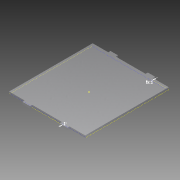
# Autodesk Inventor part: TopPanel
Saved by Autodesk Inventor 2015 SP1 (Build 190203100, 203)
## iProperties
Created: 2015-01-22
Part Number: TopPanel
Material: Acrylic, Clear
Document SubType Name: Modeling
Designer: Patrick
Density: 1.19 g/cm^3
Appearance: Transparent - Clear
Author: Patrick
Autodesk Inventor part; units mm, degrees
ref_plane "YZ Plane" through (0, 0, 0) normal (1, 0, 0) x (0, 1, 0)
ref_plane "XZ Plane" through (0, 0, 0) normal (0, 1, 0) x (-1, 0, 0)
sketch "Sketch1" plane through (0, 0, 0) normal (0, 0, 1) x (1, 0, 0)
  line L0 (-51, 56) -> (51, 56)
  line L1 (51, 56) -> (51, -56)
  line L2 (51, -56) -> (-51, -56)
  line L3 (-51, -56) -> (-51, 56)
  line L4 (-51, 56) -> (51, -56) construction
  line L5 (51, 56) -> (-51, -56) construction
  point P0 (0, 0)
  point P1 (0, 0)
  point P2 (0, 0)
  dimension "d0" = 102
  dimension "d1" = 112
  constraints: 12 end point, 3 midpoint, 2 parallel, 1 coincident, 1 horizontal, 1 perpendicular
  measures "d0" distance of L1.end L2.end
  measures "d1" distance of L0.end L1.end
extrude "Extrusion1" add sketch "Sketch1" along normal blind 3
sketch "Sketch2" plane through (0, 0, 3) normal (0, 0, 1) x (1, 0, 0)
  line L0 (-51, -56) -> (51, -56) projected
  line L1 (-30.065, -59) -> (-19.935, -59)
  line L2 (-19.935, -59) -> (-19.935, -56)
  line L3 (-19.935, -56) -> (-30.065, -56)
  line L4 (-30.065, -56) -> (-30.065, -59)
  line L5 (-30.065, -59) -> (-19.935, -56) construction
  line L6 (-19.935, -59) -> (-30.065, -56) construction
  line L7 (19.935, -59) -> (30.065, -59)
  line L8 (30.065, -59) -> (30.065, -56)
  line L9 (30.065, -56) -> (19.935, -56)
  line L10 (19.935, -56) -> (19.935, -59)
  line L11 (19.935, -59) -> (30.065, -56) construction
  line L12 (30.065, -59) -> (19.935, -56) construction
  point P0 (0, 0)
  point P1 (-25, -57.5)
  point P2 (25, -57.5)
  dimension "d4" = 3
  dimension "d5" = 25
  dimension "d6" = 25
  dimension "d7" = 10.13
  dimension "d8" = 10.13
  constraints: 24 end point, 4 midpoint, 4 parallel, 2 horizontal, 2 perpendicular, 2 point on line, 1 collinear
  measures "d4" distance of L3.end L1.start
  measures "d5" horizontal distance of point (0, 0) point (-25, -57.5)
  measures "d6" horizontal distance of point (25, -57.5) point (0, 0)
  measures "d7" distance of L1.start L1.end
  measures "d8" distance of L7.start L7.end
extrude "Extrusion2" add sketch "Sketch2" against normal blind 3
mirror "Mirror1" about plane through (0, 0, 0) normal (0, 1, 0) of "Extrusion2"
sketch "Sketch3" plane through (0, 0, 0) normal (0, 0, -1) x (-1, 0, 0)
  line L0 (-51, -56) -> (-51, 56) construction
  line L1 (-51, 55) -> (51, 55) construction
  line L2 (51, 56) -> (51, -56) construction
  line L3 (-51, -55) -> (51, -55) construction
  line L4 (-19.935, -56) -> (19.935, -56) construction
  line L5 (-30.065, 56) -> (-51, 56) construction
  point P0 (0, 0)
  dimension "d11" = 1
  dimension "d12" = 1
  constraints: 4 end point, 4 point on line, 1 horizontal, 1 perpendicular
  measures "d11" distance between parallel lines of L4 L3
  measures "d12" distance between parallel lines of L5 L1
ref_plane "Work Plane1" through (-19.935, -55, 0) normal (0, -1, 0) x (1, 0, 0)
sketch "Sketch6" plane through (0, 0, 3) normal (0, 0, 1) x (1, 0, 0)
  line L0 (30.065, -56) -> (51, -56) projected
  line L1 (51, -56) -> (51, 56) projected
  point P0 (0, 0)
  point P1 (20.6, -36.4)
  dimension "d41" = 19.6
  dimension "d42" = 30.4
  measures "d41" distance from line of L0 point (20.6, -36.4)
  measures "d42" distance from line of L1 point (20.6, -36.4)
hole "Hole4" [suppressed]
pattern_linear "Rectangular Pattern1" [suppressed]
sketch "Sketch7" plane through (0, 0, 3) normal (0, 0, 1) x (1, 0, 0)
  spline S0 degree 3 poles (-17.7549, 22.0592) (-20.3586, 22.7486) (-27.8891, 27.7258) (-21.8129, 49.2984) knots 3 3 3 3 4 4 4 4
  line L0 (-20.3586, 22.7486) -> (-27.8891, 27.7258) construction
  line L1 (-17.7549, 22.0592) -> (-20.3586, 22.7486) construction
  line L2 (-27.8891, 27.7258) -> (-21.8129, 49.2984) construction
  spline S1 degree 3 poles (-35.4301, 25.2372) (-34.47, 24.8476) (-28.6027, 22.0592) (-17.7549, 22.0592) knots 2 2 2 2 3 3 3 3
  line L3 (-35.4301, 25.2372) -> (-34.47, 24.8476) construction
  line L4 (-34.47, 24.8476) -> (-28.6027, 22.0592) construction
  line L5 (-28.6027, 22.0592) -> (-17.7549, 22.0592) construction
  spline S2 degree 3 poles (-41.3451, 44.549) (-42.3928, 42.443) (-47.2601, 32.6596) (-35.4301, 25.2372) knots 1 1 1 1 2 2 2 2
  line L6 (-41.3451, 44.549) -> (-42.3928, 42.443) construction
  line L7 (-42.3928, 42.443) -> (-47.2601, 32.6596) construction
  line L8 (-47.2601, 32.6596) -> (-35.4301, 25.2372) construction
  spline S3 degree 3 poles (-37.458, 43.3832) (-40.0894, 43.0815) (-41.2381, 43.3832) (-41.3451, 44.549) knots 0 0 0 0 1 1 1 1
  line L9 (-40.0894, 43.0815) -> (-41.2381, 43.3832) construction
  line L10 (-37.458, 43.3832) -> (-40.0894, 43.0815) construction
  line L11 (-41.2381, 43.3832) -> (-41.3451, 44.549) construction
  spline S4 degree 3 poles (-21.8129, 49.2984) (-21.8202, 49.2933) (-29.1299, 44.232) (-37.458, 43.3832) knots 4 4 4 4 5 5 5 5
  line L12 (-21.8129, 49.2984) -> (-29.1299, 44.232) construction
  line L13 (-29.1299, 44.232) -> (-37.458, 43.3832) construction
  spline S5 degree 3 poles (-15.7483, 21.8123) (-16.0581, 21.8979) (-29.0611, 22.4788) (-21.0119, 50.2568) knots 3 3 3 3 4 4 4 4
  line L14 (-15.7483, 21.8123) -> (-16.0581, 21.8979) construction
  line L15 (-16.0581, 21.8979) -> (-29.0611, 22.4788) construction
  line L16 (-29.0611, 22.4788) -> (-21.0119, 50.2568) construction
  spline S6 degree 3 poles (-21.0119, 50.2568) (-21.2194, 50.1207) (-29.151, 44.9225) (-36.6832, 43.8886) knots 4 4 4 4 5 5 5 5
  line L17 (-21.0119, 50.2568) -> (-21.2194, 50.1207) construction
  line L18 (-21.2194, 50.1207) -> (-29.151, 44.9225) construction
  line L19 (-29.151, 44.9225) -> (-36.6832, 43.8886) construction
  line L20 (-36.6832, 43.8886) -> (-35.9502, 47.0532)
  spline S7 degree 3 poles (-35.9502, 47.0532) (-35.9625, 47.0497) (-40.7954, 45.8307) (-41.6808, 44.7755) knots 0 0 0 0 1 1 1 1
  line L21 (-35.9502, 47.0532) -> (-35.9625, 47.0497) construction
  line L22 (-35.9625, 47.0497) -> (-40.7954, 45.8307) construction
  line L23 (-40.7954, 45.8307) -> (-41.6808, 44.7755) construction
  spline S8 degree 3 poles (-41.6808, 44.7755) (-41.6808, 44.7755) (-49.0375, 32.8716) (-35.5714, 24.8043) knots 1 1 1 1 2 2 2 2
  line L24 (-41.6808, 44.7755) -> (-41.6808, 44.7755) construction
  line L25 (-41.6808, 44.7755) -> (-49.0375, 32.8716) construction
  line L26 (-49.0375, 32.8716) -> (-35.5714, 24.8043) construction
  spline S9 degree 3 poles (-35.5714, 24.8043) (-35.5511, 24.7921) (-28.5456, 20.8762) (-15.7483, 21.8123) knots 2 2 2 2 3 3 3 3
  line L27 (-35.5714, 24.8043) -> (-35.5511, 24.7921) construction
  line L28 (-35.5511, 24.7921) -> (-28.5456, 20.8762) construction
  line L29 (-28.5456, 20.8762) -> (-15.7483, 21.8123) construction
  line L30 (-15.2682, 33.8195) -> (-22.3387, 33.8195) construction
  line L31 (-22.3387, 33.8195) -> (-22.3387, 39.2773) construction
  line L32 (-22.3387, 39.2773) -> (-15.2682, 39.2773) construction
  line L33 (-15.2682, 39.2773) -> (-15.2682, 33.8195) construction
  line L34 (-24.7016, 33.8748) -> (-43.5687, 33.8748) construction
  line L35 (-43.5687, 33.8748) -> (-43.5687, 39.6523) construction
  line L36 (-43.5687, 39.6523) -> (-24.7016, 39.6523) construction
  line L37 (-24.7016, 39.6523) -> (-24.7016, 33.8748) construction
  line L38 (-13.4408, 37.5513) -> (-45.6182, 37.5513) construction
  spline S10 degree 3 poles (38.6981, -46.4393) (32.5457, -44.8102) (14.7509, -33.0491) (29.1091, 17.9269) knots 3 3 3 3 4 4 4 4
  line L39 (38.6981, -46.4393) -> (32.5457, -44.8102) construction
  line L40 (32.5457, -44.8102) -> (14.7509, -33.0491) construction
  line L41 (14.7509, -33.0491) -> (29.1091, 17.9269) construction
  spline S11 degree 3 poles (-3.0683, -38.9296) (-0.7996, -39.8503) (13.0647, -46.4393) (38.6981, -46.4393) knots 2 2 2 2 3 3 3 3
  line L42 (-3.0683, -38.9296) -> (-0.7996, -39.8503) construction
  line L43 (-0.7996, -39.8503) -> (13.0647, -46.4393) construction
  line L44 (13.0647, -46.4393) -> (38.6981, -46.4393) construction
  spline S12 degree 3 poles (-17.0455, 6.7041) (-19.5213, 1.7277) (-31.0226, -21.3906) (-3.0683, -38.9296) knots 1 1 1 1 2 2 2 2
  line L45 (-17.0455, 6.7041) -> (-19.5213, 1.7277) construction
  line L46 (-19.5213, 1.7277) -> (-31.0226, -21.3906) construction
  line L47 (-31.0226, -21.3906) -> (-3.0683, -38.9296) construction
  spline S13 degree 3 poles (-7.8603, 3.9492) (-14.0782, 3.2364) (-16.7927, 3.9492) (-17.0455, 6.7041) knots 0 0 0 0 1 1 1 1
  line L48 (-7.8603, 3.9492) -> (-14.0782, 3.2364) construction
  line L49 (-14.0782, 3.2364) -> (-16.7927, 3.9492) construction
  line L50 (-16.7927, 3.9492) -> (-17.0455, 6.7041) construction
  spline S14 degree 3 poles (29.1091, 17.9269) (29.0918, 17.9149) (11.819, 5.9549) (-7.8603, 3.9492) knots 4 4 4 4 5 5 5 5
  line L51 (29.1091, 17.9269) -> (11.819, 5.9549) construction
  line L52 (11.819, 5.9549) -> (-7.8603, 3.9492) construction
  spline S15 degree 3 poles (43.4399, -47.0227) (42.7078, -46.8204) (11.9815, -45.4479) (31.0019, 20.1915) knots 3 3 3 3 4 4 4 4
  line L53 (43.4399, -47.0227) -> (42.7078, -46.8204) construction
  line L54 (42.7078, -46.8204) -> (11.9815, -45.4479) construction
  line L55 (11.9815, -45.4479) -> (31.0019, 20.1915) construction
  spline S16 degree 3 poles (31.0019, 20.1915) (30.5115, 19.8701) (11.7692, 7.5867) (-6.0293, 5.1437) knots 4 4 4 4 5 5 5 5
  line L56 (31.0019, 20.1915) -> (30.5115, 19.8701) construction
  line L57 (30.5115, 19.8701) -> (11.7692, 7.5867) construction
  line L58 (11.7692, 7.5867) -> (-6.0293, 5.1437) construction
  line L59 (-6.0293, 5.1437) -> (-4.2974, 12.6214)
  spline S17 degree 3 poles (-4.2974, 12.6214) (-4.3264, 12.6132) (-15.7465, 9.7327) (-17.8388, 7.2392) knots 0 0 0 0 1 1 1 1
  line L60 (-4.2974, 12.6214) -> (-4.3264, 12.6132) construction
  line L61 (-4.3264, 12.6132) -> (-15.7465, 9.7327) construction
  line L62 (-15.7465, 9.7327) -> (-17.8388, 7.2392) construction
  spline S18 degree 3 poles (-17.8388, 7.2392) (-17.8388, 7.2392) (-35.2226, -20.8896) (-3.4022, -39.9527) knots 1 1 1 1 2 2 2 2
  line L63 (-17.8388, 7.2392) -> (-17.8388, 7.2392) construction
  line L64 (-17.8388, 7.2392) -> (-35.2226, -20.8896) construction
  line L65 (-35.2226, -20.8896) -> (-3.4022, -39.9527) construction
  spline S19 degree 3 poles (-3.4022, -39.9527) (-3.3542, -39.9815) (13.1998, -49.2348) (43.4399, -47.0227) knots 2 2 2 2 3 3 3 3
  line L66 (-3.4022, -39.9527) -> (-3.3542, -39.9815) construction
  line L67 (-3.3542, -39.9815) -> (13.1998, -49.2348) construction
  line L68 (13.1998, -49.2348) -> (43.4399, -47.0227) construction
  line L69 (44.5744, -18.6497) -> (27.8666, -18.6497) construction
  line L70 (27.8666, -18.6497) -> (27.8666, -5.753) construction
  line L71 (27.8666, -5.753) -> (44.5744, -5.753) construction
  line L72 (44.5744, -5.753) -> (44.5744, -18.6497) construction
  line L73 (22.2831, -18.519) -> (-22.2999, -18.519) construction
  line L74 (-22.2999, -18.519) -> (-22.2999, -4.8668) construction
  line L75 (-22.2999, -4.8668) -> (22.2831, -4.8668) construction
  line L76 (22.2831, -4.8668) -> (22.2831, -18.519) construction
  line L77 (48.8924, -17.3822) -> (-27.1429, -9.8315) construction
  point P0 (0, 0)
  point P1 (-46.1734, 35.5024)
  point P2 (-28.4547, -14.6731)
  point P3 (36.4717, -44.6082)
  point P4 (32.5457, -41.4669)
  point P5 (29.1091, -36.761)
  point P6 (27.1695, -32.4025)
  point P7 (25.7734, -27.2321)
  point P8 (24.9854, -21.3562)
  point P9 (24.7959, -14.6712)
  point P10 (25.3026, -6.9857)
  point P11 (26.1472, -0.3981)
  point P12 (27.414, 5.5982)
  point P13 (28.9178, 11.9055)
  point P14 (23.0904, 15.6216)
  point P15 (16.165, 12.2433)
  point P16 (8.2261, 8.9495)
  point P17 (0.7095, 6.6692)
  point P18 (-13.648, 9.5407)
  point P19 (-20.2241, 2.0414)
  point P20 (-22.4199, -6.8265)
  point P21 (-21.9132, -16.5389)
  point P22 (-18.6194, -25.4913)
  point P23 (-13.721, -31.9099)
  point P24 (-8.4465, -36.7937)
  point P25 (-1.1832, -41.0165)
  point P26 (7.0934, -43.888)
  point P27 (14.1878, -45.4927)
  point P28 (21.8732, -46.6751)
  point P29 (34.6261, -47.3507)
  point P30 (28.2919, -47.1818)
  point P31 (-5.2552, 8.4859)
  point P32 (-13.2219, 3.7788)
  point P33 (-8.6285, 11.4147)
  point P34 (-16.5626, 5.2105)
  point P35 (-9.2199, 3.595)
  constraints: 10 end point, 9 coincident, 5 point on line, 76 other
hole "Hole5" [suppressed]
equation "\"d6\" = d5"
equation "\"d8\" = d7"
equation "\"d12\" = d11"
equation "\"kerf\" = 0.13"
body "Solid1"
